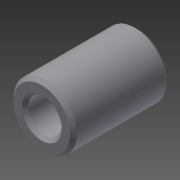
# Autodesk Inventor part: BearingLinearLMU10
Saved by Autodesk Inventor 2016 (Build 200138000, 138)
## iProperties
Category: Hardware
Created: 2014-08-22
Part Number: BearingLinearLMU10
Material: Generic
Document SubType Name: Modeling
Designer: t_clevj
Density: 1 g/cm^3
Appearance: Default
Mass: 5.85357 g
Surface Area: 29.4532 cm^2
Volume: 5.85357 cm^3
Vendor: Misumi
Catalog Web Link: http://us.misumi-ec.com/vona2/detail/110300026540/
Author: t_clevj
Title: Bearing Linear LMU10
Autodesk Inventor part; units mm, degrees
ref_plane "YZ Plane" through (0, 0, 0) normal (1, 0, 0) x (0, 1, 0)
ref_plane "XZ Plane" through (0, 0, 0) normal (0, 1, 0) x (-1, 0, 0)
ref_plane "XY Plane" through (0, 0, 0) normal (0, 0, 1) x (1, 0, 0)
sketch "Sketch1" plane through (0, 0, 0) normal (0, 1, 0) x (-1, 0, 0)
  circle A0 centre (0, 0) radius 5
  circle A1 centre (0, 0) radius 9.5
  dimension "d0" = 10
  dimension "d1" = 19
  constraints: 2 centre point, 2 coincident
  measures "d0" diameter of A0
  measures "d1" diameter of A1
extrude "Extrusion1" add sketch "Sketch1" along normal blind 29
chamfer "Chamfer1" distance 1 angle 45 4 edges at (9.5, 29, 0) (9.5, 0, 0) (5, 29, 0) (5, 0, 0)
body "Solid1"
